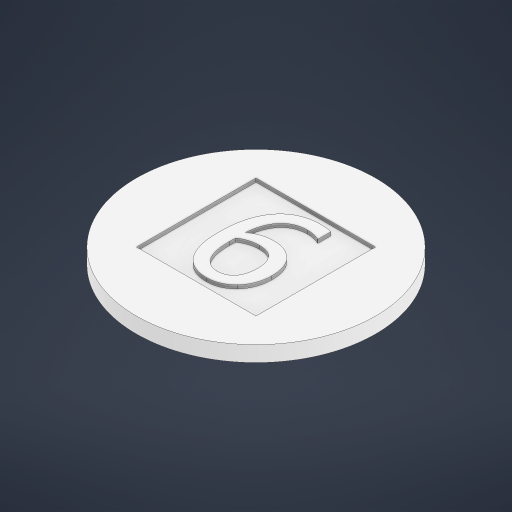
# Autodesk Inventor part: TopMarker1
Saved by Autodesk Inventor 2023.2 (Build 272271030, 271C)
## iProperties
Created: 2023-03-04
Part Number: TopMarker1
Material: Generic
Document SubType Name: Modeling
Designer: Elias Braun
Density: 1 g/cm^3
Appearance: Default
Author: Elias Braun
Autodesk Inventor part; units mm, degrees
ref_plane "YZ Plane" through (0, 0, 0) normal (1, 0, 0) x (0, 1, 0)
ref_plane "XZ Plane" through (0, 0, 0) normal (0, 1, 0) x (-1, 0, 0)
ref_plane "XY Plane" through (0, 0, 0) normal (0, 0, 1) x (1, 0, 0)
sketch "Sketch1" plane through (0, 0, 0) normal (0, 1, 0) x (-1, 0, 0)
  circle A0 centre (0, 0) radius 20
  dimension "d0" = 40
  constraints: 1 centre point, 1 coincident
  measures "d0" diameter of A0
extrude "Extrusion1" add sketch "Sketch1" along normal blind 2.6
sketch "Sketch2" plane through (0, 2.6, 0) normal (0, 1, 0) x (1, 0, 0)
  line L0 (10, -10) -> (-10, -10)
  line L1 (-10, -10) -> (-10, 10)
  line L2 (-10, 10) -> (10, 10)
  line L3 (10, 10) -> (10, -10)
  line L4 (10, -10) -> (-10, 10) construction
  line L5 (-10, -10) -> (10, 10) construction
  point P0 (0, 0)
  dimension "d3" = 20
  dimension "d4" = 20
  constraints: 12 end point, 2 midpoint, 2 parallel, 1 horizontal, 1 perpendicular
  measures "d3" distance of L0.start L0.end
  measures "d4" distance of L0.end L1.end
extrude "Extrusion2" cut sketch "Sketch2" against normal blind 0.6
sketch "Sketch4" plane through (0, 2, 0) normal (0, 1, 0) x (1, 0, 0)
  line L0 (-6.2199, 8.694) -> (6.2369, 8.694) construction
  line L1 (6.2369, 8.694) -> (6.2369, -8.5651) construction
  line L2 (6.2369, -8.5651) -> (-6.2199, -8.5651) construction
  line L3 (-6.2199, -8.5651) -> (-6.2199, 8.694) construction
  spline S0 degree 2 poles (5.4835, -2.8345) (5.4835, -4.1124) (4.6361, -6.2782) (3.9231, -7.0047) knots 0 0 0 1 2 2 2
  spline S1 degree 2 poles (3.9231, -7.0047) (3.1832, -7.7714) (1.3268, -8.5651) (0.2103, -8.5651) knots 0 0 0 1 2 2 2
  spline S2 degree 2 poles (0.2103, -8.5651) (-0.9062, -8.5651) (-2.7492, -7.8118) (-3.4487, -7.0585) knots 0 0 0 1 2 2 2
  spline S3 degree 2 poles (-3.4487, -7.0585) (-4.3096, -6.1572) (-5.2782, -3.1304) (-5.2782, -0.9243) knots 0 0 0 1 2 2 2
  spline S4 degree 2 poles (-5.2782, -0.9243) (-5.2782, 1.2415) (-4.3904, 4.7256) (-3.4622, 6.0171) knots 0 0 0 1 2 2 2
  spline S5 degree 2 poles (-3.4622, 6.0171) (-2.5609, 7.2816) (0.291, 8.694) (2.1609, 8.694) knots 0 0 0 1 2 2 2
  spline S6 degree 2 poles (2.1609, 8.694) (2.7124, 8.694) (3.681, 8.5864) (4.0442, 8.4654) knots 0 0 0 1 2 2 2
  line L4 (4.0442, 8.4654) -> (4.0442, 6.3265)
  line L5 (4.0442, 6.3265) -> (3.95, 6.3265)
  spline S7 degree 2 poles (3.95, 6.3265) (3.6406, 6.4879) (2.5106, 6.7704) (1.8649, 6.7704) knots 0 0 0 1 2 2 2
  spline S8 degree 2 poles (1.8649, 6.7704) (-0.2067, 6.7704) (-2.7492, 3.9723) (-2.9913, 1.2281) knots 0 0 0 1 2 2 2
  spline S9 degree 2 poles (-2.9913, 1.2281) (-2.1977, 1.7796) (-0.5296, 2.385) (0.4659, 2.385) knots 0 0 0 1 2 2 2
  spline S10 degree 2 poles (0.4659, 2.385) (1.4344, 2.385) (2.8873, 1.9949) (3.681, 1.403) knots 0 0 0 1 2 2 2
  spline S11 degree 2 poles (3.681, 1.403) (4.5957, 0.7169) (5.4835, -1.4085) (5.4835, -2.8345) knots 0 0 0 1 2 2 2
  spline S12 degree 2 poles (3.2236, -2.9286) (3.2236, -1.9063) (2.6855, -0.5207) (2.0936, -0.0364) knots 0 0 0 1 2 2 2
  spline S13 degree 2 poles (2.0936, -0.0364) (1.6497, 0.3133) (0.5466, 0.542) (-0.0319, 0.542) knots 0 0 0 1 2 2 2
  spline S14 degree 2 poles (-0.0319, 0.542) (-0.8121, 0.542) (-2.2784, 0.0712) (-2.9913, -0.3727) knots 0 0 0 1 2 2 2
  spline S15 degree 2 poles (-2.9913, -0.3727) (-3.0048, -0.6149) (-3.0317, -1.0722) (-3.0317, -1.422) knots 0 0 0 1 2 2 2
  spline S16 degree 2 poles (-3.0317, -1.422) (-3.0317, -3.1439) (-2.3591, -5.2559) (-1.8479, -5.8074) knots 0 0 0 1 2 2 2
  spline S17 degree 2 poles (-1.8479, -5.8074) (-1.3771, -6.332) (-0.3547, -6.7491) (0.2237, -6.7491) knots 0 0 0 1 2 2 2
  spline S18 degree 2 poles (0.2237, -6.7491) (1.569, -6.7491) (3.2236, -4.8389) (3.2236, -2.9286) knots 0 0 0 1 2 2 2
  point P0 (0, 0)
  constraints: 2 other
extrude "Extrusion4" add sketch "Sketch4" along normal blind 0.6
body "Solid1"
